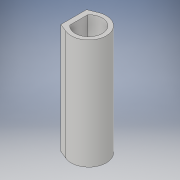
# Autodesk Inventor part: MirrorMount
Saved by Autodesk Inventor 2017 (Build 210142000, 142)
## iProperties
Created: 2017-03-28
Part Number: MirrorMount
Material: Generic
Document SubType Name: Modeling
Designer: adthune
Density: 1 g/cm^3
Appearance: Default
Author: adthune
Autodesk Inventor part; units mm, degrees
ref_plane "YZ Plane" through (0, 0, 0) normal (1, 0, 0) x (0, 1, 0)
ref_plane "XZ Plane" through (0, 0, 0) normal (0, 1, 0) x (-1, 0, 0)
ref_plane "XY Plane" through (0, 0, 0) normal (0, 0, 1) x (1, 0, 0)
sketch "Sketch1" plane through (0, 0, 0) normal (0, 1, 0) x (-1, 0, 0)
  arc A0 (2, 1.5) -> (2, -1.5) centre (0, 0) ccw
  line L0 (2, 0) -> (2, -1.5)
  line L1 (2, 0) -> (2, 1.5)
  constraints: 4 end point, 2 point on circle, 1 centre point, 1 coincident, 1 point on line, 1 vertical
sketch "Sketch1 outline for Extrusion1" plane through (0, 0, 0) normal (0, 1, 0) x (-1, 0, 0)
  line L0 (2, 0) -> (2, -1.5)
  arc A0 (2, -1.5) -> (2, 1.5) centre (0, 0) cw
  line L1 (2, 1.5) -> (2, 0)
extrude "Extrusion1" add sketch "Sketch1 outline for Extrusion1" along normal blind 22
thicken "Thicken1" operation add thickness 1 both sides no extend neighbours yes toward (-0.5598596, 0, 0.8285875) faces at (-1.399649, 14.666667, 2.071469) (-2, 14.666667, -0.5) (-2, 14.666667, 1)
sketch "Sketch2" plane through (0, 22, 0) normal (0, 1, 0) x (1, 0, 0)
  arc A0 (-2, -1.813836) -> (-2, 1.813836) centre (0, 0) ccw
  line L0 (-2, 0) -> (-2, 1.813836)
  line L1 (-2, 0) -> (-2, -1.813836)
  dimension "d8" = 5.4
  constraints: 4 end point, 2 point on circle, 1 centre point, 1 coincident, 1 point on line
  measures "d8" diameter of A0
sketch "Sketch2 outline for Extrusion2" plane through (0, 22, 0) normal (0, 1, 0) x (1, 0, 0)
  line L0 (-2, 0) -> (-2, 1.813836)
  arc A0 (-2, 1.813836) -> (-2, -1.813836) centre (0, 0) cw
  line L1 (-2, -1.813836) -> (-2, 0)
extrude "Extrusion2" cut sketch "Sketch2 outline for Extrusion2" against normal blind 22
sketch "Sketch3" plane through (0, 22, 0) normal (0, 1, 0) x (1, 0, 0)
  arc A0 (-3, -1.802776) -> (-3, 1.802776) centre (0, 0) ccw
  line L0 (-3, -1.802776) -> (-3, 2.552776)
  line L1 (-3, 2.552776) -> (-1.3277, 3.238397)
  line L2 (-3, -1.802776) -> (-3, -2.552776)
  line L3 (-3, -2.552776) -> (-1.3277, -3.238397)
  line L4 (-1.3277, -3.238397) -> (-2, -1.813836)
  line L5 (-2, 1.813836) -> (-2, -1.813836)
  line L6 (-2, -1.813836) -> (-2, 1.813836)
  line L7 (-2, 1.813836) -> (-1.3277, 3.238397)
  dimension "d12" = 4.35555
  dimension "d13" = 0.75
  constraints: 14 end point, 2 point on circle, 2 tangent, 1 collinear, 1 point on line, 1 vertical
  measures "d12" distance of L0.start L0.end
  measures "d13" distance of L0.start L2.end
sketch "Sketch3 outline for Extrusion3" plane through (0, 22, 0) normal (0, 1, 0) x (1, 0, 0)
  line L0 (-3, -2.552776) -> (-1.3277, -3.238397)
  line L1 (-1.3277, -3.238397) -> (-2, -1.813836)
  line L2 (-2, -1.813836) -> (-2, 1.813836)
  line L3 (-2, 1.813836) -> (-1.3277, 3.238397)
  line L4 (-1.3277, 3.238397) -> (-3, 2.552776)
  line L5 (-3, 2.552776) -> (-3, -2.552776)
extrude "Extrusion3" add sketch "Sketch3 outline for Extrusion3" against normal blind 22
body "Solid1"
